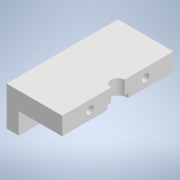
# Autodesk Inventor part: 15_Base_Dietro
Saved by Autodesk Inventor 2020 (Build 240168000, 168)
## iProperties
Created: 2019-10-17
Part Number: 15_Base_Dietro
Material: Generico
Document SubType Name: Modeling
Designer: socci
Density: 1 g/cm^3
Appearance: Default
Author: socci
Autodesk Inventor part; units mm, degrees
ref_plane "YZ Plane" through (0, 0, 0) normal (1, 0, 0) x (0, 1, 0)
ref_plane "XZ Plane" through (0, 0, 0) normal (0, 1, 0) x (-1, 0, 0)
ref_plane "XY Plane" through (0, 0, 0) normal (0, 0, 1) x (1, 0, 0)
sketch "Schizzo1" plane through (0, 0, 0) normal (0, 1, 0) x (-1, 0, 0)
  line L0 (25, 50) -> (-25, 50)
  line L1 (-25, 50) -> (-25, -50)
  line L2 (-25, -50) -> (25, -50)
  line L3 (25, -50) -> (25, 50)
  line L4 (25, 50) -> (-25, -50) construction
  line L5 (-25, 50) -> (25, -50) construction
  point P0 (0, 0)
  point P1 (0, 0)
  point P2 (0, 0)
  dimension "d0" = 50
  dimension "d9" = 100
  constraints: 12 end point, 3 midpoint, 2 parallel, 1 coincident, 1 horizontal, 1 perpendicular
  measures "d0" distance of L0.start L0.end
  measures "d9" distance of L2.end L0.start
extrude "Estrusione1" add sketch "Schizzo1" along normal blind 16
sketch "Schizzo2" plane through (0, 0, 0) normal (0, -1, 0) x (1, 0, 0)
  circle A0 centre (25, 0) radius 9.5
  line L0 (25, 50) -> (25, -50) projected
  point P0 (0, 0)
  dimension "d3" = 19
  constraints: 1 centre point, 1 coincident, 1 midpoint
  measures "d3" diameter of A0
extrude "Estrusione2" cut sketch "Schizzo2" against normal blind 4
sketch "Schizzo4" plane through (0, 4, 0) normal (0, -1, 0) x (1, 0, 0)
  circle A0 centre (25, 0) radius 6
  line L0 (25, 9.5) -> (25, -9.5) projected
  point P0 (0, 0)
  point P1 (25, 6)
  point P2 (25, -6)
  dimension "d6" = 12
  constraints: 1 centre point, 1 coincident, 1 midpoint
  measures "d6" diameter of A0
extrude "Estrusione3" cut sketch "Schizzo4" against normal blind 26 contours L0 A0 picked at (23.13, -0.7092)
sketch "Schizzo5" plane through (-25, 0, -50) normal (-1, 0, 0) x (0, 0, 1)
  line L0 (50, 0) -> (50, 8)
  line L1 (50, 8) -> (75, 8)
  line L2 (50, 8) -> (25, 8)
  line L3 (50, 8) -> (75, 8) construction
  dimension "d10" = 8
  dimension "d11" = 25
  dimension "d12" = 25
  dimension "d13" = 180
  constraints: 8 end point, 2 horizontal, 1 collinear, 1 perpendicular, 1 vertical
  measures "d10" distance of L0.start L0.end
  measures "d11" distance of L0.end L1.end
  measures "d12" distance of L0.end L2.end
  measures "d13" angle of L2 L3
hole "Foro1" at (-25, 8, -25) at (-25, 8, 25) direction (1, 0, 0) diameter 6.6 end through all clearance for "Bullone a testa esagonale" size "M6" standard "ANSI - Profilo M Metrico"
sketch "Schizzo6" plane through (-25, 0, -50) normal (-1, 0, 0) x (0, 0, 1)
  circle A0 centre (25, 8) radius 3.3 projected
  circle A1 centre (25, 8) radius 5
  circle A2 centre (75, 8) radius 3.3 projected
  circle A3 centre (75, 8) radius 5
  circle A4 centre (25, 8) radius 3.3 projected
  line L0 (27.8868, 13) -> (30.7735, 8)
  line L1 (30.7735, 8) -> (27.8868, 3)
  line L2 (27.8868, 3) -> (22.1132, 3)
  line L3 (22.1132, 3) -> (19.2265, 8)
  line L4 (19.2265, 8) -> (22.1132, 13)
  line L5 (22.1132, 13) -> (27.8868, 13)
  line L6 (77.8868, 13) -> (80.7735, 8)
  line L7 (80.7735, 8) -> (77.8868, 3)
  line L8 (77.8868, 3) -> (72.1132, 3)
  line L9 (72.1132, 3) -> (69.2265, 8)
  line L10 (69.2265, 8) -> (72.1132, 13)
  line L11 (72.1132, 13) -> (77.8868, 13)
  point P0 (50, 0)
  point P1 (25, 13)
  point P2 (75, 13)
  dimension "d21" = 10
  dimension "d22" = 10
  constraints: 24 end point, 4 coincident, 2 midpoint, 2 vertical alignment, 1 point on line, 31 other
extrude "Estrusione4" cut sketch "Schizzo6" against normal blind 6 contours A0 | A1 | A1 L0 L1 | A1 L5 L0 | L1 L2 A1 | A1 L4 L5 | L2 L3 A1 | A1 L3 L4 | A2 | A3 | A3 L6 L7 | A3 L11 L6 | L7 L8 A3 | A3 L10 L11 | L8 L9 A3 | A3 L9 L10
